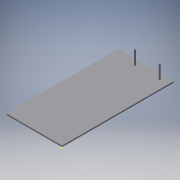
# Autodesk Inventor part: base
Saved by Autodesk Inventor 2019 (Build 230136000, 136)
## iProperties
Created: 2018-07-24
Part Number: base
Material: Genérico
Document SubType Name: Modeling
Designer: Ernandes
Density: 1 g/cm^3
Appearance: Padrão
Author: Ernandes
Autodesk Inventor part; units mm, degrees
ref_plane "YZ Plane" through (0, 0, 0) normal (1, 0, 0) x (0, 1, 0)
ref_plane "XZ Plane" through (0, 0, 0) normal (0, 1, 0) x (-1, 0, 0)
ref_plane "XY Plane" through (0, 0, 0) normal (0, 0, 1) x (1, 0, 0)
sketch "Esboço1" plane through (0, 0, 0) normal (0, 1, 0) x (-1, 0, 0)
  point P0 (0, 0)
sketch "Esboço2" plane through (0, 0, 0) normal (0, 1, 0) x (-1, 0, 0)
  line L0 (0, 0) -> (0, -400)
  line L1 (0, -400) -> (200, -400)
  line L2 (200, -400) -> (200, 0)
  line L3 (200, 0) -> (0, 0)
  dimension "d0" = 400
  dimension "d1" = 200
  constraints: 8 end point, 3 perpendicular, 1 vertical
  measures "d0" distance of L0.start L0.end
  measures "d1" distance of L0.end L1.end
extrude "Extrusão1" add sketch "Esboço2" along normal blind 5
sketch "Esboço3" plane through (0, 0, 0) normal (1, 0, 0) x (0, 0, -1)
  point P0 (0, 0)
sketch "Esboço4" plane through (0, 5, 0) normal (0, 1, 0) x (1, 0, 0)
  line L0 (-32.5, 380) -> (-32.5, 382.5)
  line L1 (-32.5, 382.5) -> (-27.5, 382.5)
  line L2 (-27.5, 382.5) -> (-27.5, 377.5)
  line L3 (-27.5, 377.5) -> (-32.5, 377.5)
  line L4 (-32.5, 377.5) -> (-32.5, 380)
  line L5 (-122.0302, 380) -> (-122.0302, 382.5)
  line L6 (-122.0302, 382.5) -> (-117.0302, 382.5)
  line L7 (-117.0302, 382.5) -> (-117.0302, 377.5)
  line L8 (-117.0302, 377.5) -> (-122.0302, 377.5)
  line L9 (-122.0302, 377.5) -> (-122.0302, 380)
  point P0 (0, 0)
  constraints: 20 end point, 8 perpendicular, 2 point on line, 2 vertical
extrude "Extrusão3" add sketch "Esboço4" along normal blind 30
sketch "Esboço5" plane through (-27.5, 5, -382.5) normal (0, 0, -1) x (-1, 0, 0)
  line L0 (0, 0) -> (0, 30) projected
  line L1 (5, 0) -> (5, 30) projected
  line L2 (0, 30) -> (5, 30)
  line L3 (5, 30) -> (5, 25.0023)
  line L4 (5, 25.0023) -> (0, 25.0023)
  line L5 (0, 25.0023) -> (0, 30)
  line L6 (89.5302, 0) -> (89.5302, 30) projected
  line L7 (94.5302, 0) -> (94.5302, 30) projected
  line L8 (89.5302, 30) -> (94.5302, 30)
  line L9 (94.5302, 30) -> (94.5302, 25.0023)
  line L10 (94.5302, 25.0023) -> (89.5302, 25.0023)
  line L11 (89.5302, 25.0023) -> (89.5302, 30)
  point P0 (-27.5, -5)
  constraints: 16 end point, 4 parallel, 3 point on line, 2 horizontal, 2 perpendicular
extrude "Extrusão4" add sketch "Esboço5" along normal blind 20
fillet "Arredondamento1" radius 2 21 edges at (-27.5, 32.5011, -402.5) (-27.5, 35, -390) (-30, 35, -402.5) (-32.5, 32.5011, -402.5) (-30, 30.0023, -402.5) (-27.5, 30.0023, -392.5) (-32.5, 35, -390) (-27.5, 20, -377.5) (-27.5, 17.5011, -382.5) (-32.5, 17.5011, -382.5) (-117.0302, 17.5011, -382.5) (-117.0302, 20, -377.5) (-122.0302, 35, -390) (-117.0302, 35, -390) (-117.0302, 32.5011, -402.5) (-119.5302, 30.0023, -402.5) (-117.0302, 30.0023, -392.5) (-122.0302, 32.5011, -402.5) (-122.0302, 17.5011, -382.5) (-32.5, 20, -377.5) (-122.0302, 20, -377.5)
